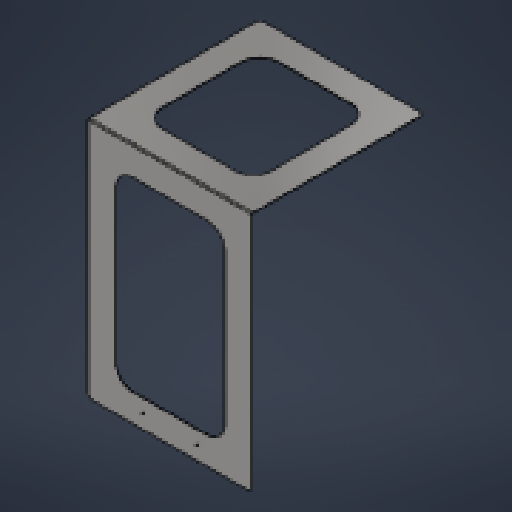
# Autodesk Inventor part: Side Panel
Saved by Autodesk Inventor 2026 (Build 300175050, 175E)
## iProperties
Created: 2025-05-19
Part Number: Side Panel
Material: Steel, Carbon
Document SubType Name: Sheet Metal
Designer: Joshua Eah
Density: 7.85 g/cm^3
Sheet Metal Rule: A36 Steel 20 ga
Appearance: Semi-Polished
Author: Joshua Eah
Autodesk Inventor part; units mm, degrees
ref_plane "YZ Plane" through (0, 0, 0) normal (1, 0, 0) x (0, 1, 0)
ref_plane "XZ Plane" through (0, 0, 0) normal (0, 1, 0) x (-1, 0, 0)
ref_plane "XY Plane" through (0, 0, 0) normal (0, 0, 1) x (1, 0, 0)
sketch "Sketch1" plane through (0, 0, 0) normal (0, 1, 0) x (-1, 0, 0)
  line L0 (0, 0) -> (-230, 0)
  line L1 (-230, 0) -> (-230, -337.35)
  line L2 (-230, -337.35) -> (0, -337.35)
  line L3 (0, -337.35) -> (0, 0)
  line L4 (-115, -337.35) -> (-115, 0) construction
  line L5 (-38.1, -299.25) -> (-191.9, -299.25)
  line L6 (-191.9, -299.25) -> (-191.9, -38.1)
  line L7 (-191.9, -38.1) -> (-38.1, -38.1)
  line L8 (-38.1, -38.1) -> (-38.1, -299.25)
  line L9 (-38.1, -299.25) -> (-191.9, -38.1) construction
  line L10 (-191.9, -299.25) -> (-38.1, -38.1) construction
  circle A0 centre (-76.9, -19.05) radius 1.6
  circle A1 centre (-153.1, -19.05) radius 1.6
  point P0 (-115, -168.675)
  dimension "d0" = 230
  dimension "d1" = 337.35
  dimension "d18" = 38.1
  dimension "d20" = 38.1
  dimension "d21" = 38.1
  dimension "d59" = 3.2
  dimension "d60" = 19.05
  dimension "d61" = 76.2
  dimension "d62" = 38.1
  measures "d0" distance of L2.end L1.end
  measures "d1" distance of L1.end L0.end
  measures "d18" distance between parallel lines of L2 L5
  measures "d20" distance between parallel lines of L0 L7
  measures "d21" distance between parallel lines of L3 L8
  measures "d59" diameter of A0
  measures "d60" distance from line of L0 A0.centre
  measures "d61" distance of A1.centre A0.centre
  measures "d62" distance from line of A0.centre L4
extrude "Plate3" add sketch "Sketch1" along normal blind 0.9119
sketch "Sketch4" plane through (230, -0.9119, -338.2619) normal (0, 0, -1) x (-1, 0, 0)
  line L0 (230, 0) -> (0, 0)
  line L1 (0, 0) -> (0, -239.35)
  line L2 (0, -239.35) -> (230, -239.35)
  line L3 (230, -239.35) -> (230, 0)
  constraints: 6 end point, 1 horizontal, 1 perpendicular, 1 vertical
edge flange "Flange2" height 241.1737 angle 90 thickness 0.9119 bend radius 0.9119 thickness toward (0, 0, -1) relief straight relief width 0.9119 relief depth 0.4559 edges at (115, 0, -337.35) wall of the first edge with corners at (0, -0.9119, -338.2619) (230, -0.9119, -338.2619) (230, -240.2619, -338.2619) (0, -240.2619, -338.2619)
bend "Bend2"
corner "Corner2"
unfold all bends "Unfold2" k factor 0.44 fixed face at (12.7, 0.9119, -212.2)
sketch "Sketch5" plane through (0, 0.9119, -578.7626) normal (0, 1, 0) x (1, 0, 0)
  line L0 (0, -239.35) -> (230, -239.35) projected
  line L1 (230, 0) -> (230, -239.35) projected
  line L2 (0, 0) -> (230, 0) projected
  line L3 (0, -239.35) -> (0, 0) projected
  line L4 (38.1, -38.1) -> (191.9, -38.1)
  line L5 (191.9, -38.1) -> (191.9, -201.25)
  line L6 (191.9, -201.25) -> (38.1, -201.25)
  line L7 (38.1, -201.25) -> (38.1, -38.1)
  point P0 (0, -578.7626)
  dimension "d52" = 38.1
  dimension "d53" = 38.1
  dimension "d54" = 38.1
  dimension "d55" = 38.1
  constraints: 8 end point, 2 parallel, 1 horizontal, 1 perpendicular
  measures "d52" distance between parallel lines of L3 L7
  measures "d53" distance between parallel lines of L0 L6
  measures "d54" distance between parallel lines of L1 L5
  measures "d55" distance between parallel lines of L4 L2
extrude "Extrusion2" cut sketch "Sketch5" against normal through all contours L4 L5 L6 L7
refold all bends "Refold2"
fillet "Corner Round5" radius 6.35 4 edges at (230, 0.4559, 0) (0, 0.4559, 0) (230, -240.2619, -338.7178) (0, -240.2619, -338.7178)
fillet "Corner Round5" radius 25.4 8 edges at (38.1, 0.4559, -299.25) (191.9, 0.4559, -299.25) (38.1, 0.4559, -38.1) (191.9, 0.4559, -38.1) (191.9, -39.0119, -338.7178) (38.1, -39.0119, -338.7178) (38.1, -202.1619, -338.7178) (191.9, -202.1619, -338.7178)
equation "\"d20\" = d18"
equation "\"d21\" = d20"
equation "\"d62\" = 0.5 * d61"
equation "\"d53\" = d52"
equation "\"d54\" = d52"
equation "\"d55\" = d52"
equation "\"d40\" = Thickness"
equation "\"d41\" = BendReliefWidth"
equation "\"d42\" = BendReliefDepth"
equation "\"d43\" = MinimumRemnant"
equation "\"d44\" = TransitionRadius"
equation "\"d47\" = BendRadius"
equation "\"d48\" = CornerReliefSize"
equation "\"d49\" = GapSize"
equation "\"d50\" = JacobiRadiusSize"
equation "\"BendRadius\" = Thickness"
equation "\"BendReliefWidth\" = Thickness"
equation "\"BendReliefDepth\" = 0.5 * Thickness"
equation "\"CornerReliefSize\" = 4 * Thickness"
equation "\"MinimumRemnant\" = 2 * Thickness"
equation "\"TransitionRadius\" = BendRadius"
equation "\"JacobiRadiusSize\" = BendRadius"
equation "\"GapSize\" = Thickness"
equation "\"FoamThickness\" = 3"
equation "\"InsulationThickness\" = 6.35"
equation "\"Thickness\" = 0.91186"
body "Solid2"
